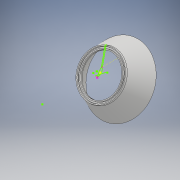
# Autodesk Inventor part: A1V1M2_dropArm_superWOK_tall_interface_FULL_360
Saved by Autodesk Inventor 2018 (Build 220112000, 112)
## iProperties
Created: 2018-04-20
Part Number: A1V1M2_dropArm_superWOK_tall_interface_FULL_360
Material: Generic
Document SubType Name: Modeling
Designer: McCormick Lab
Density: 1 g/cm^3
Appearance: Default
Author: McCormick Lab
Autodesk Inventor part; units mm, degrees
ref_plane "YZ Plane" through (0, 0, 0) normal (1, 0, 0) x (0, 1, 0)
ref_plane "XZ Plane" through (0, 0, 0) normal (0, 1, 0) x (-1, 0, 0)
ref_plane "XY Plane" through (0, 0, 0) normal (0, 0, 1) x (1, 0, 0)
sketch "Sketch68" plane through (0, 0, 0) normal (1, 0, 0) x (0, 1, 0)
  line L0 (1, 4.6737) -> (23, 4.6737) construction
  line L1 (7.0021, -2.9903) -> (-7.0029, -0.0135)
  line L2 (7.2385, 26.8729) -> (5.7713, 27.1847)
  line L3 (2.4565, 4.3755) -> (1, 4.6737)
  line L4 (5.7713, 27.1847) -> (1, 4.6737)
  line L5 (7.2385, 26.8729) -> (2.4565, 4.3755)
  point P0 (0, 0)
  point P1 (2.225, 5.1772)
  constraints: 12 end point, 1 horizontal
sketch "Sketch184" plane through (0, 0, 0) normal (1, 0, 0) x (0, 1, 0)
  arc A0 (-3.5, -3.0972) -> (0, -1.6204) centre (-4.281, 3.6397) ccw
  arc A1 (0, -1.6204) -> (2.2822, 2) centre (-4.3557, 3.6547) ccw
  arc A2 (2.2822, 2) -> (2.459, 4.3851) centre (-8.8285, 4.0231) ccw
  arc A3 (2.459, 4.3851) -> (2.3883, 6) centre (-72.7121, 1.9029) ccw
  line L0 (-3.5, -3.0972) -> (-3.5, -3.6807) projected
  arc A4 (2.3883, 6) -> (-3.5, -3.0972) centre (8.6947, -4.5362) ccw
  point P0 (0, 0)
  constraints: 10 point on circle, 5 centre point
sketch "Sketch213" plane through (0, 0, 0) normal (1, 0, 0) x (0, 1, 0)
  line L0 (13.3414, -11.8728) -> (-10.8201, 5)
  line L1 (46.9769, 13.1952) -> (18.0214, 18.2633)
  line L2 (-13.3385, -26.1425) -> (0.7357, -50.4491)
  line L3 (0.7357, -50.4491) -> (1.9473, -49.7476)
  line L4 (1.9473, -49.7476) -> (-11.7207, -26.1425)
  line L5 (-11.7207, -26.1425) -> (-10, -24)
  line L6 (46.5114, 10.5356) -> (18.0034, 15.5254)
  line L7 (18.0034, 15.5254) -> (16.7759, 13.7195)
  line L8 (16.7759, 13.7195) -> (15.6891, 14.4784)
  line L9 (46.9769, 13.1952) -> (46.5114, 10.5356)
  line L10 (-13.3385, -26.1425) -> (-16, -24)
  line L11 (-16, -24) -> (-15.3672, -23.2139)
  line L12 (-15.3672, -23.2139) -> (-13.3385, -24.8471)
  line L13 (-13.3385, -24.8471) -> (-12.3402, -23.607)
  line L14 (-12.3402, -23.607) -> (-14.3528, -21.9897)
  line L15 (-14.3528, -21.9897) -> (-13.6273, -21.0868)
  line L16 (-10, -24) -> (-13.6273, -21.0868)
  line L17 (15.6891, 14.4784) -> (13.7085, 15.7292)
  line L18 (13.7085, 15.7292) -> (14.325, 16.7055)
  line L19 (14.325, 16.7055) -> (15.9169, 15.7001)
  line L20 (18.0214, 18.2633) -> (15.9169, 19.2263)
  line L21 (15.9169, 15.7001) -> (16.9692, 17.0103)
  line L22 (16.9692, 17.0103) -> (15.4765, 18.2639)
  line L23 (15.4765, 18.2639) -> (15.9169, 19.2263)
  point P0 (0, 0)
  point P1 (3.3399, -2.2736)
  point P2 (-1.2043, -8.7808)
  dimension "d600" = 1.4
  dimension "d601" = 2.7
  constraints: 48 end point, 1 perpendicular
  measures "d600" distance of L2.end L3.end
  measures "d601" distance of L1.start L6.start
revolve "Revolution5" add sketch "Sketch213" angle 360 about axis through (0, 13.3414, -11.8728) along (0, -0.8199, 0.5725) contours L9 L6 L7 L8 L17 L18 L19 L21 L22 L23 L20 L1
body "Solid2"
